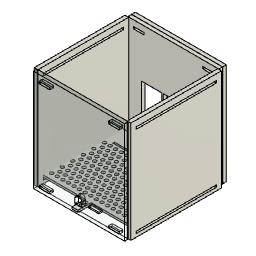
behavior box (Autodesk Fusion 360 design; units mm, degrees)
Autodesk Fusion 360 part; units mm, degrees
note: some values were not read from the file. Set by a fixed rule: the direction of a hole.
sketch "Sketch1" plane through (0, 0, 0) normal (1, 0, 0) x (0, 1, 0)
  line L0 (-7.9883, 4.5929) -> (-0.555, 4.5929)
  line L1 (-0.555, 4.5929) -> (-0.555, -3.7203)
  line L2 (-0.555, -3.7203) -> (-7.9883, -3.7203)
  line L3 (-7.9883, -3.7203) -> (-7.9883, 4.5929)
  line L4 (-7.5336, -3.2867) -> (-0.9801, -3.2867)
  line L5 (-0.9801, -3.2867) -> (-0.9801, -3.4535)
  line L6 (-0.9801, -3.4535) -> (-7.5336, -3.4535)
  line L7 (-7.5336, -3.4535) -> (-7.5336, -3.2867)
  line L8 (-7.5465, 4.1066) -> (-0.9801, 4.1066)
  line L9 (-0.9801, 4.1066) -> (-0.9801, 3.9332)
  line L10 (-0.9801, 3.9332) -> (-7.5465, 3.9332)
  line L11 (-7.5465, 3.9332) -> (-7.5465, 4.1066)
  constraint horizontal L0
  constraint vertical L1
  constraint horizontal L2
  constraint vertical L3
  constraint horizontal L4
  constraint vertical L5
  constraint horizontal L6
  constraint vertical L7
  constraint horizontal L8
  constraint vertical L9
  constraint horizontal L10
  constraint vertical L11
extrude "Extrude1" add sketch "Sketch1" along normal blind 0.3 makes body 1
move_body "Move1" bodies 1 to x (1, 0, 0) y (0, 1, 0) z (0, 0, 1) at (-7.7244, 20, 0.114)
copy_body "CopyPasteBodies1" bodies 1 makes body 2
move_body "Move2" bodies 2 to x (1, 0, 0) y (0, 1, 0) z (0, 0, 1) at (11.7466, 0.1876, -0.142)
sketch "Sketch2" plane through (0, 0, 0) normal (0, 0, 1) x (1, 0, 0)
  line L0 (-8.0919, 3.9069) -> (-0.6475, 3.9069)
  line L1 (-0.6475, 3.9069) -> (-0.6475, -2.6445)
  line L2 (-0.6475, -2.6445) -> (-8.0919, -2.6445)
  line L3 (-8.0919, -2.6445) -> (-8.0919, 3.9069)
  line L4 (-4.54, -2.6445) -> (-4.0525, -2.6445)
  line L5 (-4.0525, -2.6445) -> (-4.0525, -3.7265)
  line L6 (-4.0525, -3.7265) -> (-4.54, -3.7265)
  line L7 (-4.54, -3.7265) -> (-4.54, -2.6445)
  circle A0 centre (-4.3, -2.8685) radius 0.1404
  circle A1 centre (-4.3178, -3.2428) radius 0.1002
  line L8 (-7.3807, 2.6) -> (-1.4, 2.6)
  line L9 (-1.4, 2.6) -> (-1.4, 2.4711)
  line L10 (-1.4, 2.4711) -> (-7.3807, 2.4711)
  line L11 (-7.3807, 2.4711) -> (-7.3807, 2.6)
  line L12 (-6.1257, 3.8) -> (-6.2257, 3.8)
  line L13 (-6.2257, 3.8) -> (-6.2257, 2.9257)
  line L14 (-6.2257, 2.9257) -> (-6.1257, 2.9257)
  line L15 (-6.1257, 2.9257) -> (-6.1257, 3.8)
  line L16 (-4.4615, 3.8) -> (-4.3321, 3.8)
  line L17 (-4.3321, 3.8) -> (-4.3321, 2.9321)
  line L18 (-4.3321, 2.9321) -> (-4.4615, 2.9321)
  line L19 (-4.4615, 2.9321) -> (-4.4615, 3.8)
  line L20 (-2.6294, 3.7936) -> (-2.5155, 3.7936)
  line L21 (-2.5155, 3.7936) -> (-2.5155, 2.9257)
  line L22 (-2.5155, 2.9257) -> (-2.6294, 2.9257)
  line L23 (-2.6294, 2.9257) -> (-2.6294, 3.7936)
  constraint horizontal L0
  constraint vertical L1
  constraint horizontal L2
  constraint vertical L3
  constraint horizontal L4
  constraint vertical L5
  constraint horizontal L6
  constraint vertical L7
  constraint coincident L2 L4.start
  constraint horizontal L8
  constraint vertical L9
  constraint horizontal L10
  constraint vertical L11
  constraint horizontal L12
  constraint vertical L13
  constraint horizontal L14
  constraint vertical L15
  constraint horizontal L16
  constraint vertical L17
  constraint horizontal L18
  constraint vertical L19
  constraint horizontal L20
  constraint vertical L21
  constraint horizontal L22
  constraint vertical L23
extrude "Extrude2" add sketch "Sketch2" along normal blind 0.16 separate body makes body 3
sketch "Sketch3" plane through (0, 0, 0) normal (0, 0, 1) x (1, 0, 0)
  circle A0 centre (-7.7614, 2.1643) radius 0.1338
  circle A1 centre (-7.3065, 2.1643) radius 0.1204
  circle A2 centre (-6.8381, 2.1643) radius 0.1204
  circle A3 centre (-6.3832, 2.1643) radius 0.1265
  circle A4 centre (-5.9223, 2.1643) radius 0.1382
  circle A5 centre (-5.4723, 2.1643) radius 0.1382
  circle A6 centre (-5.013, 2.1587) radius 0.1273
  circle A7 centre (-4.5567, 2.1587) radius 0.1325
  circle A8 centre (-4.1005, 2.1623) radius 0.1376
  circle A9 centre (-3.6425, 2.1623) radius 0.135
  circle A10 centre (-3.1792, 2.1623) radius 0.135
  circle A11 centre (-2.7232, 2.1622) radius 0.135
  circle A12 centre (-2.2676, 2.1637) radius 0.1337
  circle A13 centre (-1.8117, 2.1637) radius 0.1286
  circle A14 centre (-1.3497, 2.1637) radius 0.1261
  circle A15 centre (-1.1257, 1.7247) radius 0.135
  circle A16 centre (-1.5848, 1.7237) radius 0.1327
  circle A17 centre (-2.0357, 1.7237) radius 0.1258
  circle A18 centre (-2.4977, 1.7237) radius 0.1316
  circle A19 centre (-2.9502, 1.7237) radius 0.1289
  circle A20 centre (-3.4109, 1.7237) radius 0.1317
  circle A21 centre (-3.8693, 1.7237) radius 0.1318
  circle A22 centre (-4.3227, 1.7237) radius 0.1334
  circle A23 centre (-4.7836, 1.7237) radius 0.1306
  circle A24 centre (-5.2425, 1.7237) radius 0.1329
  circle A25 centre (-5.697, 1.7237) radius 0.1287
  circle A26 centre (-6.1519, 1.7237) radius 0.1351
  circle A27 centre (-6.6125, 1.7407) radius 0.1274
  circle A28 centre (-7.0636, 1.7407) radius 0.1234
  circle A29 centre (-7.5313, 1.7274) radius 0.1318
  dimension "d6" = 0.27
  dimension "d7" = 0.27
  dimension "d8" = 0.27
  measures "d6" diameter of A10
  measures "d7" diameter of A11
  measures "d8" diameter of A15
hole "Hole1" at (-7.7538, 2.1618, 0.16) direction (0, 0, -1) diameter 0.27 depth 0.3 tip angle 118 bodies 3
hole "Hole2" at (-7.3065, 2.1643, 0) direction (0, 0, 1) diameter 0.27 depth 0.16 tip angle 118 bodies 3
hole "Hole3" at (-6.8421, 2.1458, 0.16) direction (0, 0, -1) diameter 0.27 depth 0.16 tip angle 118 bodies 3
hole "Hole4" at (-6.3808, 2.1692, 0.16) direction (0, 0, -1) diameter 0.27 depth 0.16 tip angle 118 bodies 3
hole "Hole5" at (-5.9263, 2.1659, 0.16) direction (0, 0, -1) diameter 0.27 depth 0.16 tip angle 118 bodies 3
hole "Hole6" at (-5.4673, 2.1644, 0.16) direction (0, 0, -1) diameter 0.27 depth 0.16 tip angle 118 bodies 3
hole "Hole7" at (-5.0162, 2.1602, 0.16) direction (0, 0, -1) diameter 0.27 depth 0.16 tip angle 118 bodies 3
hole "Hole8" at (-4.7761, 1.7189, 0.16) direction (0, 0, -1) diameter 0.27 depth 0.16 tip angle 118 bodies 3
hole "Hole9" at (-5.0058, 1.3054, 0.16) direction (0, 0, -1) diameter 0.27 depth 0.16 tip angle 118 bodies 3
hole "Hole10" at (-4.5547, 2.1575, 0.16) direction (0, 0, -1) diameter 0.27 depth 0.16 tip angle 118 bodies 3
hole "Hole11" at (-4.1036, 2.1658, 0.16) direction (0, 0, -1) diameter 0.27 depth 0.16 tip angle 118 bodies 3
hole "Hole12" at (-3.6316, 2.1575, 0.16) direction (0, 0, -1) diameter 0.27 depth 0.16 tip angle 118 bodies 3
hole "Hole13" at (-3.1827, 2.1742, 0.16) direction (0, 0, -1) diameter 0.27 depth 0.16 tip angle 118 bodies 3
hole "Hole14" at (-2.7256, 2.1587, 0.16) direction (0, 0, -1) diameter 0.27 depth 0.16 tip angle 118 bodies 3
hole "Hole15" at (-2.2693, 2.1536, 0.16) direction (0, 0, -1) diameter 0.27 depth 0.16 tip angle 118 bodies 3
hole "Hole16" at (-1.8021, 2.1536, 0.16) direction (0, 0, -1) diameter 0.27 depth 0.16 tip angle 118 bodies 3
hole "Hole17" at (-1.3481, 2.158, 0.16) direction (0, 0, -1) diameter 0.27 depth 0.16 tip angle 118 bodies 3
hole "Hole18" at (-1.1189, 1.7217, 0.16) direction (0, 0, -1) diameter 0.27 depth 0.16 tip angle 118 bodies 3
hole "Hole19" at (-1.5729, 1.7261, 0.16) direction (0, 0, -1) diameter 0.27 depth 0.16 tip angle 118 bodies 3
hole "Hole20" at (-2.0401, 1.7261, 0.16) direction (0, 0, -1) diameter 0.27 depth 0.16 tip angle 118 bodies 3
hole "Hole21" at (-2.4941, 1.7217, 0.16) direction (0, 0, -1) diameter 0.27 depth 0.16 tip angle 118 bodies 3
hole "Hole22" at (-2.948, 1.7261, 0.16) direction (0, 0, -1) diameter 0.27 depth 0.16 tip angle 118 bodies 3
hole "Hole23" at (-3.4064, 1.7261, 0.16) direction (0, 0, -1) diameter 0.27 depth 0.16 tip angle 118 bodies 3
hole "Hole24" at (-1.8073, 1.2873, 0.16) direction (0, 0, -1) diameter 0.27 depth 0.16 tip angle 118 bodies 3
hole "Hole25" at (-1.3504, 1.2921, 0.16) direction (0, 0, -1) diameter 0.27 depth 0.16 tip angle 118 bodies 3
hole "Hole26" at (-2.2671, 1.2965, 0.16) direction (0, 0, -1) diameter 0.27 depth 0.16 tip angle 118 bodies 3
hole "Hole27" at (-2.7255, 1.2921, 0.16) direction (0, 0, -1) diameter 0.27 depth 0.16 tip angle 118 bodies 3
hole "Hole28" at (-1.1167, 0.8513, 0.16) direction (0, 0, -1) diameter 0.27 depth 0.16 tip angle 118 bodies 3
hole "Hole29" at (-1.5796, 0.8645, 0.16) direction (0, 0, -1) diameter 0.27 depth 0.16 tip angle 118 bodies 3
hole "Hole30" at (-2.0379, 0.8601, 0.16) direction (0, 0, -1) diameter 0.27 depth 0.16 tip angle 118 bodies 3
hole "Hole31" at (-2.4963, 0.8645, 0.16) direction (0, 0, -1) diameter 0.27 depth 0.16 tip angle 118 bodies 3
hole "Hole32" at (-1.3504, 0.4149, 0.16) direction (0, 0, -1) diameter 0.27 depth 0.16 tip angle 118 bodies 3
hole "Hole33" at (-1.8176, 0.437, 0.16) direction (0, 0, -1) diameter 0.27 depth 0.16 tip angle 118 bodies 3
hole "Hole34" at (-2.2627, 0.4282, 0.16) direction (0, 0, -1) diameter 0.27 depth 0.16 tip angle 118 bodies 3
hole "Hole35" at (-3.8747, 1.7287, 0.16) direction (0, 0, -1) diameter 0.27 depth 0.16 tip angle 118 bodies 3
hole "Hole36" at (-3.1867, 1.2953, 0.16) direction (0, 0, -1) diameter 0.27 depth 0.16 tip angle 118 bodies 3
hole "Hole37" at (-3.4103, 0.855, 0.16) direction (0, 0, -1) diameter 0.27 depth 0.16 tip angle 118 bodies 3
hole "Hole38" at (-2.9527, 0.8653, 0.16) direction (0, 0, -1) diameter 0.27 depth 0.16 tip angle 118 bodies 3
hole "Hole39" at (-2.7223, 0.4215, 0.16) direction (0, 0, -1) diameter 0.27 depth 0.16 tip angle 118 bodies 3
hole "Hole40" at (-3.1867, 0.4318, 0.16) direction (0, 0, -1) diameter 0.27 depth 0.16 tip angle 118 bodies 3
hole "Hole41" at (-3.6408, 1.2981, 0.16) direction (0, 0, -1) diameter 0.27 depth 0.16 tip angle 118 bodies 3
hole "Hole42" at (-3.8718, 0.8556, 0.16) direction (0, 0, -1) diameter 0.27 depth 0.16 tip angle 118 bodies 3
hole "Hole43" at (-3.6375, 0.4326, 0.16) direction (0, 0, -1) diameter 0.27 depth 0.16 tip angle 118 bodies 3
hole "Hole44" at (-3.4065, -0.0132, 0.16) direction (0, 0, -1) diameter 0.27 depth 0.16 tip angle 118 bodies 3
hole "Hole45" at (-2.9575, -0.0001, 0.16) direction (0, 0, -1) diameter 0.27 depth 0.16 tip angle 118 bodies 3
hole "Hole46" at (-2.4922, -0.0132, 0.16) direction (0, 0, -1) diameter 0.27 depth 0.16 tip angle 118 bodies 3
hole "Hole47" at (-2.0302, -0.0099, 0.16) direction (0, 0, -1) diameter 0.27 depth 0.16 tip angle 118 bodies 3
hole "Hole48" at (-1.5774, -0.0094, 0.16) direction (0, 0, -1) diameter 0.27 depth 0.16 tip angle 118 bodies 3
hole "Hole49" at (-1.1208, -0.0027, 0.16) direction (0, 0, -1) diameter 0.27 depth 0.16 tip angle 118 bodies 3
hole "Hole50" at (-1.3474, -0.4459, 0.16) direction (0, 0, -1) diameter 0.27 depth 0.16 tip angle 118 bodies 3
hole "Hole51" at (-1.8073, -0.4459, 0.16) direction (0, 0, -1) diameter 0.27 depth 0.16 tip angle 118 bodies 3
hole "Hole52" at (-2.2638, -0.4392, 0.16) direction (0, 0, -1) diameter 0.27 depth 0.16 tip angle 118 bodies 3
hole "Hole53" at (-2.717, -0.4359, 0.16) direction (0, 0, -1) diameter 0.27 depth 0.16 tip angle 118 bodies 3
hole "Hole54" at (-3.1802, -0.4392, 0.16) direction (0, 0, -1) diameter 0.27 depth 0.16 tip angle 118 bodies 3
hole "Hole55" at (-1.1164, -0.8803, 0.16) direction (0, 0, -1) diameter 0.27 depth 0.16 tip angle 118 bodies 3
hole "Hole56" at (-1.5814, -0.8755, 0.16) direction (0, 0, -1) diameter 0.27 depth 0.16 tip angle 118 bodies 3
hole "Hole57" at (-2.0272, -0.8707, 0.16) direction (0, 0, -1) diameter 0.27 depth 0.16 tip angle 118 bodies 3
hole "Hole58" at (-2.497, -0.8707, 0.16) direction (0, 0, -1) diameter 0.27 depth 0.16 tip angle 118 bodies 3
hole "Hole59" at (-2.9524, -0.8803, 0.16) direction (0, 0, -1) diameter 0.27 depth 0.16 tip angle 118 bodies 3
hole "Hole60" at (-1.3417, -1.3117, 0.16) direction (0, 0, -1) diameter 0.27 depth 0.16 tip angle 118 bodies 3
hole "Hole61" at (-1.8019, -1.3165, 0.16) direction (0, 0, -1) diameter 0.27 depth 0.16 tip angle 118 bodies 3
hole "Hole62" at (-2.2621, -1.3117, 0.16) direction (0, 0, -1) diameter 0.27 depth 0.16 tip angle 118 bodies 3
hole "Hole63" at (-2.7175, -1.3117, 0.16) direction (0, 0, -1) diameter 0.27 depth 0.16 tip angle 118 bodies 3
hole "Hole64" at (-3.1777, -1.3165, 0.16) direction (0, 0, -1) diameter 0.27 depth 0.16 tip angle 118 bodies 3
hole "Hole65" at (-3.4078, -0.8803, 0.16) direction (0, 0, -1) diameter 0.27 depth 0.16 tip angle 118 bodies 3
hole "Hole66" at (-3.6427, -0.4441, 0.16) direction (0, 0, -1) diameter 0.27 depth 0.16 tip angle 118 bodies 3
hole "Hole67" at (-3.8776, -0.003, 0.16) direction (0, 0, -1) diameter 0.27 depth 0.16 tip angle 118 bodies 3
hole "Hole68" at (-4.0933, -0.4441, 0.16) direction (0, 0, -1) diameter 0.27 depth 0.16 tip angle 118 bodies 3
hole "Hole69" at (-3.8657, -0.8824, 0.16) direction (0, 0, -1) diameter 0.27 depth 0.16 tip angle 118 bodies 3
hole "Hole70" at (-4.0958, 0.4263, 0.16) direction (0, 0, -1) diameter 0.27 depth 0.16 tip angle 118 bodies 3
hole "Hole71" at (-4.3211, -0.0147, 0.16) direction (0, 0, -1) diameter 0.27 depth 0.16 tip angle 118 bodies 3
hole "Hole72" at (-4.556, 0.4311, 0.16) direction (0, 0, -1) diameter 0.27 depth 0.16 tip angle 118 bodies 3
hole "Hole73" at (-4.7861, -0.0003, 0.16) direction (0, 0, -1) diameter 0.27 depth 0.16 tip angle 118 bodies 3
hole "Hole74" at (-5.0114, 0.412, 0.16) direction (0, 0, -1) diameter 0.27 depth 0.16 tip angle 118 bodies 3
hole "Hole75" at (-4.5464, -0.4365, 0.16) direction (0, 0, -1) diameter 0.27 depth 0.16 tip angle 118 bodies 3
hole "Hole76" at (-5.0114, -0.4413, 0.16) direction (0, 0, -1) diameter 0.27 depth 0.16 tip angle 118 bodies 3
hole "Hole77" at (-4.7717, -0.8776, 0.16) direction (0, 0, -1) diameter 0.27 depth 0.16 tip angle 118 bodies 3
hole "Hole78" at (-4.3211, -0.868, 0.16) direction (0, 0, -1) diameter 0.27 depth 0.16 tip angle 118 bodies 3
hole "Hole79" at (-3.6256, -1.3146, 0.16) direction (0, 0, -1) diameter 0.27 depth 0.16 tip angle 118 bodies 3
hole "Hole80" at (-4.1002, -1.305, 0.16) direction (0, 0, -1) diameter 0.27 depth 0.16 tip angle 118 bodies 3
hole "Hole81" at (-4.5413, -1.305, 0.16) direction (0, 0, -1) diameter 0.27 depth 0.16 tip angle 118 bodies 3
hole "Hole82" at (-1.1137, -1.746, 0.16) direction (0, 0, -1) diameter 0.27 depth 0.16 tip angle 118 bodies 3
hole "Hole83" at (-1.5739, -1.7412, 0.16) direction (0, 0, -1) diameter 0.27 depth 0.16 tip angle 118 bodies 3
hole "Hole84" at (-2.0341, -1.7412, 0.16) direction (0, 0, -1) diameter 0.27 depth 0.16 tip angle 118 bodies 3
hole "Hole85" at (-2.4895, -1.7412, 0.16) direction (0, 0, -1) diameter 0.27 depth 0.16 tip angle 118 bodies 3
hole "Hole86" at (-2.9497, -1.7508, 0.16) direction (0, 0, -1) diameter 0.27 depth 0.16 tip angle 118 bodies 3
hole "Hole87" at (-3.4003, -1.7412, 0.16) direction (0, 0, -1) diameter 0.27 depth 0.16 tip angle 118 bodies 3
hole "Hole88" at (-3.8605, -1.7412, 0.16) direction (0, 0, -1) diameter 0.27 depth 0.16 tip angle 118 bodies 3
hole "Hole89" at (-4.3207, -1.746, 0.16) direction (0, 0, -1) diameter 0.27 depth 0.16 tip angle 118 bodies 3
hole "Hole90" at (-4.7809, -1.7364, 0.16) direction (0, 0, -1) diameter 0.27 depth 0.16 tip angle 118 bodies 3
hole "Hole91" at (-5.011, -1.3146, 0.16) direction (0, 0, -1) diameter 0.27 depth 0.16 tip angle 118 bodies 3
hole "Hole92" at (-5.2363, -0.864, 0.16) direction (0, 0, -1) diameter 0.27 depth 0.16 tip angle 118 bodies 3
hole "Hole93" at (-5.476, -1.3098, 0.16) direction (0, 0, -1) diameter 0.27 depth 0.16 tip angle 118 bodies 3
hole "Hole94" at (-5.2316, -1.7508, 0.16) direction (0, 0, -1) diameter 0.27 depth 0.16 tip angle 118 bodies 3
hole "Hole95" at (-5.4712, -0.4469, 0.16) direction (0, 0, -1) diameter 0.27 depth 0.16 tip angle 118 bodies 3
hole "Hole96" at (-5.6918, -0.8736, 0.16) direction (0, 0, -1) diameter 0.27 depth 0.16 tip angle 118 bodies 3
hole "Hole97" at (-1.803, -2.1746, 0.16) direction (0, 0, -1) diameter 0.27 depth 0.16 tip angle 118 bodies 3
hole "Hole98" at (-1.3463, -2.1743, 0.16) direction (0, 0, -1) diameter 0.27 depth 0.16 tip angle 118 bodies 3
hole "Hole99" at (-2.2635, -2.1775, 0.16) direction (0, 0, -1) diameter 0.27 depth 0.16 tip angle 118 bodies 3
hole "Hole100" at (-2.7223, -2.1723, 0.16) direction (0, 0, -1) diameter 0.27 depth 0.16 tip angle 118 bodies 3
hole "Hole101" at (-3.176, -2.1723, 0.16) direction (0, 0, -1) diameter 0.27 depth 0.16 tip angle 118 bodies 3
hole "Hole102" at (-3.6373, -2.1775, 0.16) direction (0, 0, -1) diameter 0.27 depth 0.16 tip angle 118 bodies 3
hole "Hole103" at (-4.0836, -2.1805, 0.16) direction (0, 0, -1) diameter 0.27 depth 0.16 tip angle 118 bodies 3
hole "Hole104" at (-4.5474, -2.1763, 0.16) direction (0, 0, -1) diameter 0.27 depth 0.16 tip angle 118 bodies 3
hole "Hole105" at (-5.0112, -2.1763, 0.16) direction (0, 0, -1) diameter 0.27 depth 0.16 tip angle 118 bodies 3
hole "Hole106" at (-5.9181, -1.315, 0.16) direction (0, 0, -1) diameter 0.27 depth 0.16 tip angle 118 bodies 3
hole "Hole107" at (-5.6862, -1.7415, 0.16) direction (0, 0, -1) diameter 0.27 depth 0.16 tip angle 118 bodies 3
hole "Hole108" at (-5.4709, -2.1722, 0.16) direction (0, 0, -1) diameter 0.27 depth 0.16 tip angle 118 bodies 3
hole "Hole109" at (-5.9181, -2.1722, 0.16) direction (0, 0, -1) diameter 0.27 depth 0.16 tip angle 118 bodies 3
hole "Hole110" at (-6.15, -1.7415, 0.16) direction (0, 0, -1) diameter 0.27 depth 0.16 tip angle 118 bodies 3
hole "Hole111" at (-6.3778, -2.1722, 0.16) direction (0, 0, -1) diameter 0.27 depth 0.16 tip angle 118 bodies 3
hole "Hole112" at (-6.8271, -2.1796, 0.16) direction (0, 0, -1) diameter 0.27 depth 0.16 tip angle 118 bodies 3
hole "Hole113" at (-7.2992, -2.1671, 0.16) direction (0, 0, -1) diameter 0.27 depth 0.16 tip angle 118 bodies 3
hole "Hole114" at (-7.7464, -2.1713, 0.16) direction (0, 0, -1) diameter 0.27 depth 0.16 tip angle 118 bodies 3
hole "Hole115" at (-6.6076, -1.7406, 0.16) direction (0, 0, -1) diameter 0.27 depth 0.16 tip angle 118 bodies 3
hole "Hole116" at (-7.0672, -1.7406, 0.16) direction (0, 0, -1) diameter 0.27 depth 0.16 tip angle 118 bodies 3
hole "Hole117" at (-7.5186, -1.7406, 0.16) direction (0, 0, -1) diameter 0.27 depth 0.16 tip angle 118 bodies 3
hole "Hole118" at (-6.3757, -1.3016, 0.16) direction (0, 0, -1) diameter 0.27 depth 0.16 tip angle 118 bodies 3
hole "Hole119" at (-6.8395, -1.3016, 0.16) direction (0, 0, -1) diameter 0.27 depth 0.16 tip angle 118 bodies 3
hole "Hole120" at (-7.2813, -1.3194, 0.16) direction (0, 0, -1) diameter 0.27 depth 0.16 tip angle 118 bodies 3
hole "Hole121" at (-7.7492, -1.307, 0.16) direction (0, 0, -1) diameter 0.27 depth 0.16 tip angle 118 bodies 3
hole "Hole122" at (-6.1466, -0.8721, 0.16) direction (0, 0, -1) diameter 0.27 depth 0.16 tip angle 118 bodies 3
hole "Hole123" at (-6.6104, -0.8763, 0.16) direction (0, 0, -1) diameter 0.27 depth 0.16 tip angle 118 bodies 3
hole "Hole124" at (-7.0577, -0.8721, 0.16) direction (0, 0, -1) diameter 0.27 depth 0.16 tip angle 118 bodies 3
hole "Hole125" at (-7.5215, -0.868, 0.16) direction (0, 0, -1) diameter 0.27 depth 0.16 tip angle 118 bodies 3
hole "Hole126" at (-5.9147, -0.4415, 0.16) direction (0, 0, -1) diameter 0.27 depth 0.16 tip angle 118 bodies 3
hole "Hole127" at (-6.3826, -0.4415, 0.16) direction (0, 0, -1) diameter 0.27 depth 0.16 tip angle 118 bodies 3
hole "Hole128" at (-6.8315, -0.4413, 0.16) direction (0, 0, -1) diameter 0.27 depth 0.16 tip angle 118 bodies 3
hole "Hole129" at (-7.2953, -0.4455, 0.16) direction (0, 0, -1) diameter 0.27 depth 0.16 tip angle 118 bodies 3
hole "Hole130" at (-7.7508, -0.4413, 0.16) direction (0, 0, -1) diameter 0.27 depth 0.16 tip angle 118 bodies 3
hole "Hole131" at (-7.5231, -0.0106, 0.16) direction (0, 0, -1) diameter 0.27 depth 0.16 tip angle 118 bodies 3
hole "Hole132" at (-7.0675, -0.0024, 0.16) direction (0, 0, -1) diameter 0.27 depth 0.16 tip angle 118 bodies 3
hole "Hole133" at (-6.6037, -0.0024, 0.16) direction (0, 0, -1) diameter 0.27 depth 0.16 tip angle 118 bodies 3
hole "Hole134" at (-6.144, -0.0106, 0.16) direction (0, 0, -1) diameter 0.27 depth 0.16 tip angle 118 bodies 3
hole "Hole135" at (-5.6968, -0.0065, 0.16) direction (0, 0, -1) diameter 0.27 depth 0.16 tip angle 118 bodies 3
hole "Hole136" at (-5.2288, 0.0018, 0.16) direction (0, 0, -1) diameter 0.27 depth 0.16 tip angle 118 bodies 3
hole "Hole137" at (-7.755, 0.4325, 0.16) direction (0, 0, -1) diameter 0.27 depth 0.16 tip angle 118 bodies 3
hole "Hole138" at (-7.5231, 0.8673, 0.16) direction (0, 0, -1) diameter 0.27 depth 0.16 tip angle 118 bodies 3
hole "Hole139" at (-7.2953, 1.2938, 0.16) direction (0, 0, -1) diameter 0.27 depth 0.16 tip angle 118 bodies 3
hole "Hole140" at (-7.287, 0.4407, 0.16) direction (0, 0, -1) diameter 0.27 depth 0.16 tip angle 118 bodies 3
hole "Hole141" at (-7.08, 0.859, 0.16) direction (0, 0, -1) diameter 0.27 depth 0.16 tip angle 118 bodies 3
hole "Hole142" at (-6.8356, 1.3021, 0.16) direction (0, 0, -1) diameter 0.27 depth 0.16 tip angle 118 bodies 3
hole "Hole143" at (-6.6079, 0.859, 0.16) direction (0, 0, -1) diameter 0.27 depth 0.16 tip angle 118 bodies 3
hole "Hole144" at (-6.8522, 0.4407, 0.16) direction (0, 0, -1) diameter 0.27 depth 0.16 tip angle 118 bodies 3
hole "Hole145" at (-6.3842, 0.4325, 0.16) direction (0, 0, -1) diameter 0.27 depth 0.16 tip angle 118 bodies 3
hole "Hole146" at (-5.9287, 0.4325, 0.16) direction (0, 0, -1) diameter 0.27 depth 0.16 tip angle 118 bodies 3
hole "Hole147" at (-6.1523, 0.8673, 0.16) direction (0, 0, -1) diameter 0.27 depth 0.16 tip angle 118 bodies 3
hole "Hole148" at (-5.4649, 0.42, 0.16) direction (0, 0, -1) diameter 0.27 depth 0.16 tip angle 118 bodies 3
hole "Hole149" at (-5.6844, 0.8507, 0.16) direction (0, 0, -1) diameter 0.27 depth 0.16 tip angle 118 bodies 3
hole "Hole150" at (-5.233, 0.8631, 0.16) direction (0, 0, -1) diameter 0.27 depth 0.16 tip angle 118 bodies 3
hole "Hole151" at (-4.7774, 0.859, 0.16) direction (0, 0, -1) diameter 0.27 depth 0.16 tip angle 118 bodies 3
hole "Hole152" at (-4.3219, 0.859, 0.16) direction (0, 0, -1) diameter 0.27 depth 0.16 tip angle 118 bodies 3
hole "Hole153" at (-4.0941, 1.3104, 0.16) direction (0, 0, -1) diameter 0.27 depth 0.16 tip angle 118 bodies 3
hole "Hole154" at (-4.558, 1.2938, 0.16) direction (0, 0, -1) diameter 0.27 depth 0.16 tip angle 118 bodies 3
hole "Hole155" at (-5.4607, 1.2938, 0.16) direction (0, 0, -1) diameter 0.27 depth 0.16 tip angle 118 bodies 3
hole "Hole156" at (-5.9204, 1.2855, 0.16) direction (0, 0, -1) diameter 0.27 depth 0.16 tip angle 118 bodies 3
hole "Hole157" at (-6.3718, 1.2897, 0.16) direction (0, 0, -1) diameter 0.27 depth 0.16 tip angle 118 bodies 3
hole "Hole158" at (-7.5131, 1.7234, 0.16) direction (0, 0, -1) diameter 0.27 depth 0.16 tip angle 118 bodies 3
hole "Hole159" at (-7.7657, 1.2927, 0.16) direction (0, 0, -1) diameter 0.27 depth 0.16 tip angle 118 bodies 3
hole "Hole160" at (-7.0658, 1.7192, 0.16) direction (0, 0, -1) diameter 0.27 depth 0.16 tip angle 118 bodies 3
hole "Hole161" at (-6.6103, 1.7192, 0.16) direction (0, 0, -1) diameter 0.27 depth 0.16 tip angle 118 bodies 3
hole "Hole162" at (-6.1506, 1.7234, 0.16) direction (0, 0, -1) diameter 0.27 depth 0.16 tip angle 118 bodies 3
hole "Hole163" at (-5.6965, 1.7204, 0.16) direction (0, 0, -1) diameter 0.27 depth 0.16 tip angle 118 bodies 3
hole "Hole164" at (-5.2326, 1.7163, 0.16) direction (0, 0, -1) diameter 0.27 depth 0.16 tip angle 118 bodies 3
hole "Hole165" at (-4.3174, 1.7287, 0.16) direction (0, 0, -1) diameter 0.27 depth 0.16 tip angle 118 bodies 3
move_body "Move3" bodies 3 to x (1, 0, 0) y (0, 1, 0) z (0, 0, 1) at (0.5247, 15.1211, -3.1578)
move_body "Move4" bodies 2 to x (1, 0, 0) y (0, 1, 0) z (0, 0, 1) at (-4.1588, -0.1688, 0.1425)
sketch "Sketch4" plane through (0, 0, 0) normal (0, 1, 0) x (1, 0, 0)
  line L0 (18.0903, 3.7329) -> (10.6559, 3.7329)
  line L1 (10.6559, 3.7329) -> (10.6559, -4.5899)
  line L2 (10.6559, -4.5899) -> (18.0903, -4.5899)
  line L3 (18.0903, -4.5899) -> (18.0903, 3.7329)
  line L4 (11.1, 3.2792) -> (11.9723, 3.2792)
  line L5 (11.9723, 3.2792) -> (11.9723, 3.4485)
  line L6 (11.9723, 3.4485) -> (11.1, 3.4485)
  line L7 (11.1, 3.4485) -> (11.1, 3.2792)
  line L8 (16.7862, 3.4554) -> (17.6692, 3.4554)
  line L9 (17.6692, 3.4554) -> (17.6692, 3.2792)
  line L10 (17.6692, 3.2792) -> (16.7862, 3.2792)
  line L11 (16.7862, 3.2792) -> (16.7862, 3.4554)
  line L12 (11.7551, -0.5653) -> (13.408, -0.5653)
  line L13 (13.408, -0.5653) -> (13.408, 2.3)
  line L14 (13.408, 2.3) -> (11.7551, 2.3)
  line L15 (11.7551, 2.3) -> (11.7551, -0.5653)
  line L16 (12.1551, 2.3) -> (13.0157, 2.3)
  line L17 (13.0157, 2.3) -> (13.0157, 3.6472)
  line L18 (13.0157, 3.6472) -> (12.1551, 3.6472)
  line L19 (12.1551, 3.6472) -> (12.1551, 2.3)
  line L20 (13.5394, -0.5663) -> (15.2015, -0.5663)
  line L21 (15.2015, -0.5663) -> (15.2015, 2.2924)
  line L22 (15.2015, 2.2924) -> (13.5394, 2.2924)
  line L23 (13.5394, 2.2924) -> (13.5394, -0.5663)
  line L24 (14.8, 3.6448) -> (13.9269, 3.6448)
  line L25 (13.9269, 3.6448) -> (13.9269, 2.2924)
  line L26 (13.9269, 2.2924) -> (14.8, 2.2924)
  line L27 (14.8, 2.2924) -> (14.8, 3.6448)
  line L28 (15.3552, -0.5617) -> (16.9944, -0.5617)
  line L29 (16.9944, -0.5617) -> (16.9944, 2.2924)
  line L30 (16.9944, 2.2924) -> (15.3552, 2.2924)
  line L31 (15.3552, 2.2924) -> (15.3552, -0.5617)
  line L32 (15.7344, 2.2924) -> (16.6118, 2.2924)
  line L33 (16.6118, 2.2924) -> (16.6118, 3.6471)
  line L34 (16.6118, 3.6471) -> (15.7344, 3.6471)
  line L35 (15.7344, 3.6471) -> (15.7344, 2.2924)
  line L36 (11.1, -4.1125) -> (11.9614, -4.1125)
  line L37 (11.9614, -4.1125) -> (11.9614, -3.9451)
  line L38 (11.9614, -3.9451) -> (11.1, -3.9451)
  line L39 (11.1, -3.9451) -> (11.1, -4.1125)
  line L40 (16.7794, -4.1124) -> (17.6573, -4.1124)
  line L41 (17.6573, -4.1124) -> (17.6573, -3.9391)
  line L42 (17.6573, -3.9391) -> (16.7794, -3.9391)
  line L43 (16.7794, -3.9391) -> (16.7794, -4.1124)
  constraint horizontal L0
  constraint vertical L1
  constraint horizontal L2
  constraint vertical L3
  constraint horizontal L4
  constraint vertical L5
  constraint horizontal L6
  constraint vertical L7
  constraint horizontal L8
  constraint vertical L9
  constraint horizontal L10
  constraint vertical L11
  constraint horizontal L12
  constraint vertical L13
  constraint horizontal L14
  constraint vertical L15
  constraint horizontal L16
  constraint vertical L17
  constraint horizontal L18
  constraint vertical L19
  constraint coincident L14 L16.start
  constraint horizontal L20
  constraint vertical L21
  constraint horizontal L22
  constraint vertical L23
  constraint horizontal L24
  constraint vertical L25
  constraint horizontal L26
  constraint vertical L27
  constraint coincident L22 L25.end
  constraint horizontal L28
  constraint vertical L29
  constraint horizontal L30
  constraint vertical L31
  constraint horizontal L32
  constraint vertical L33
  constraint horizontal L34
  constraint vertical L35
  constraint coincident L30 L32.start
  constraint horizontal L36
  constraint vertical L37
  constraint horizontal L38
  constraint vertical L39
  constraint horizontal L40
  constraint vertical L41
  constraint horizontal L42
  constraint vertical L43
extrude "Extrude3" add sketch "Sketch4" along normal blind 0.3 separate body makes body 4
sketch "Sketch5" plane through (0, 0, 0) normal (1, 0, 0) x (0, 1, 0)
sketch "Sketch6" plane through (0, 0, 0) normal (0, 1, 0) x (1, 0, 0)
  line L0 (28.6506, -4.5834) -> (36.1053, -4.5834)
  line L1 (36.1053, -4.5834) -> (36.1053, 3.7081)
  line L2 (36.1053, 3.7081) -> (28.6506, 3.7081)
  line L3 (28.6506, 3.7081) -> (28.6506, -4.5834)
  line L4 (29.0918, -4.1152) -> (29.9715, -4.1152)
  line L5 (29.9715, -4.1152) -> (29.9715, -3.9408)
  line L6 (29.9715, -3.9408) -> (29.0918, -3.9408)
  line L7 (29.0918, -3.9408) -> (29.0918, -4.1152)
  line L8 (34.7838, -4.113) -> (35.6579, -4.113)
  line L9 (35.6579, -4.113) -> (35.6579, -3.9421)
  line L10 (35.6579, -3.9421) -> (34.7838, -3.9421)
  line L11 (34.7838, -3.9421) -> (34.7838, -4.113)
  line L12 (29.1, 3.2832) -> (29.9664, 3.2832)
  line L13 (29.9664, 3.2832) -> (29.9664, 3.4552)
  line L14 (29.9664, 3.4552) -> (29.1, 3.4552)
  line L15 (29.1, 3.4552) -> (29.1, 3.2832)
  line L16 (34.7861, 3.2815) -> (35.663, 3.2815)
  line L17 (35.663, 3.2815) -> (35.663, 3.4584)
  line L18 (35.663, 3.4584) -> (34.7861, 3.4584)
  line L19 (34.7861, 3.4584) -> (34.7861, 3.2815)
  line L20 (29.3122, -1.1002) -> (35.4253, -1.1002)
  line L21 (35.7753, -0.7502) -> (35.7753, 2.4927)
  line L22 (35.4253, 2.8427) -> (29.3122, 2.8427)
  line L23 (28.9622, 2.4927) -> (28.9622, -0.7502)
  arc A0 (28.9622, -0.7502) -> (29.3122, -1.1002) centre (29.3122, -0.7502) ccw
  arc A1 (35.4253, -1.1002) -> (35.7753, -0.7502) centre (35.4253, -0.7502) ccw
  arc A2 (29.3122, 2.8427) -> (28.9622, 2.4927) centre (29.3122, 2.4927) ccw
  arc A3 (35.7753, 2.4927) -> (35.4253, 2.8427) centre (35.4253, 2.4927) ccw
  arc A4 (32.6691, 2.8426) -> (32.3813, 3.1428) centre (32.3687, 2.8427) ccw
  arc A5 (32.3813, 3.1428) -> (32.0684, 2.8424) centre (32.3687, 2.8427) ccw
  arc A6 (34.4813, 2.8427) -> (34.1814, 3.1494) centre (34.1745, 2.8427) ccw
  arc A7 (34.1814, 3.1494) -> (33.8678, 2.8426) centre (34.1745, 2.8427) ccw
  arc A8 (30.9021, 2.8427) -> (30.5976, 3.1507) centre (30.5941, 2.8427) ccw
  arc A9 (30.5976, 3.1507) -> (30.2861, 2.8427) centre (30.5941, 2.8427) ccw
  dimension "d506" = 0.35
  dimension "d507" = 0.35
  dimension "d508" = 0.35
  dimension "d509" = 0.35
  constraint horizontal L0
  constraint vertical L1
  constraint horizontal L2
  constraint vertical L3
  constraint horizontal L4
  constraint vertical L5
  constraint horizontal L6
  constraint vertical L7
  constraint horizontal L8
  constraint vertical L9
  constraint horizontal L10
  constraint vertical L11
  constraint horizontal L12
  constraint vertical L13
  constraint horizontal L14
  constraint vertical L15
  constraint horizontal L16
  constraint vertical L17
  constraint horizontal L18
  constraint vertical L19
  constraint horizontal L20
  constraint vertical L21
  constraint horizontal L22
  constraint vertical L23
  constraint tangent L23 A0
  constraint tangent L20 A0
  constraint tangent L20 A1
  constraint tangent L21 A1
  constraint tangent L23 A2
  constraint tangent L22 A2
  constraint tangent L22 A3
  constraint tangent L21 A3
  constraint midpoint L22 A4.centre
  constraint coincident A4.centre A5.centre
  constraint coincident L22 A6.centre
  constraint coincident A6.centre A7.centre
  constraint coincident L22 A8.centre
  constraint coincident A8.centre A9.centre
  measures "d506" radius of A0
  measures "d507" radius of A1
  measures "d508" radius of A2
  measures "d509" radius of A3
extrude "Extrude5" add sketch "Sketch6" along normal blind 0.3 separate body makes body 5
move_body "Move5" bodies 4 to x (1, 0, 0) y (0, 1, 0) z (0, 0, 1) at (-27.1889, 0, -16.6152)
move_body "Move6" bodies 4 to x (1, 0, 0) y (0, 1, 0) z (0, 0, 1) at (9.0191, 19.4801, 16.7217)
move_body "Move7" bodies 5 to x (1, 0, 0) y (0, 1, 0) z (0, 0, 1) at (-36.1767, 19.7852, 0.1174)
sketch "Sketch7" plane through (0, 0, 0) normal (0, 1, 0) x (1, 0, 0)
  line L0 (19.6, 2.7241) -> (12.1495, 2.7241)
  line L1 (12.1495, 2.7241) -> (12.1495, -5.595)
  line L2 (12.1495, -5.595) -> (19.6, -5.595)
  line L3 (19.6, -5.595) -> (19.6, 2.7241)
  line L4 (12.5883, -5.1117) -> (13.4726, -5.1117)
  line L5 (13.4726, -5.1117) -> (13.4726, -4.943)
  line L6 (13.4726, -4.943) -> (12.5883, -4.943)
  line L7 (12.5883, -4.943) -> (12.5883, -5.1117)
  line L8 (18.2816, -5.1158) -> (19.1533, -5.1158)
  line L9 (19.1533, -5.1158) -> (19.1533, -4.9368)
  line L10 (19.1533, -4.9368) -> (18.2816, -4.9368)
  line L11 (18.2816, -4.9368) -> (18.2816, -5.1158)
  line L12 (12.6, 2.2859) -> (13.4703, 2.2859)
  line L13 (13.4703, 2.2859) -> (13.4703, 2.4536)
  line L14 (13.4703, 2.4536) -> (12.6, 2.4536)
  line L15 (12.6, 2.4536) -> (12.6, 2.2859)
  line L16 (16.6141, 1.7318) -> (17.5, 1.7318)
  line L17 (17.5, 1.7318) -> (17.5, 1.8424)
  line L18 (17.5, 1.8424) -> (16.6141, 1.8424)
  line L19 (16.6141, 1.8424) -> (16.6141, 1.7318)
  line L20 (18.2824, 2.2824) -> (19.1559, 2.2824)
  line L21 (19.1559, 2.2824) -> (19.1559, 2.4549)
  line L22 (19.1559, 2.4549) -> (18.2824, 2.4549)
  line L23 (18.2824, 2.4549) -> (18.2824, 2.2824)
  line L24 (15.5235, 2.1071) -> (16.0953, 2.1071)
  line L25 (16.0953, 2.1071) -> (16.0953, 1.7024)
  line L26 (15.7953, 1.4024) -> (15.8235, 1.4024)
  line L27 (15.5235, 1.7024) -> (15.5235, 2.1071)
  arc A0 (15.5235, 1.7024) -> (15.8235, 1.4024) centre (15.8235, 1.7024) ccw
  arc A1 (15.7953, 1.4024) -> (16.0953, 1.7024) centre (15.7953, 1.7024) ccw
  dimension "d514" = 0.3
  dimension "d515" = 0.3
  constraint horizontal L0
  constraint vertical L1
  constraint horizontal L2
  constraint vertical L3
  constraint horizontal L4
  constraint vertical L5
  constraint horizontal L6
  constraint vertical L7
  constraint horizontal L8
  constraint vertical L9
  constraint horizontal L10
  constraint vertical L11
  constraint horizontal L12
  constraint vertical L13
  constraint horizontal L14
  constraint vertical L15
  constraint horizontal L16
  constraint vertical L17
  constraint horizontal L18
  constraint vertical L19
  constraint horizontal L20
  constraint vertical L21
  constraint horizontal L22
  constraint vertical L23
  constraint horizontal L24
  constraint vertical L25
  constraint horizontal L26
  constraint vertical L27
  constraint tangent L27 A0
  constraint tangent L26 A0
  constraint tangent L26 A1
  constraint tangent L25 A1
  measures "d514" radius of A0
  measures "d515" radius of A1
extrude "Extrude6" add sketch "Sketch7" along normal blind 0.3 separate body makes body 6
move_body "Move8" bodies 6 to x (1, 0, 0) y (0, 1, 0) z (0, 0, 1) at (-19.66, 11.7458, -0.9059)
